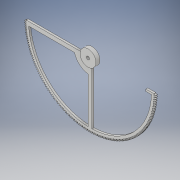
# Autodesk Inventor part: arm
Saved by Autodesk Inventor 2017 (Build 210142000, 142)
## iProperties
Created: 2016-11-23
Part Number: arm
Material: Generic
Document SubType Name: Modeling
Designer: cody
Density: 1 g/cm^3
Appearance: Default
Author: cody
Autodesk Inventor part; units mm, degrees
ref_plane "YZ Plane" through (0, 0, 0) normal (1, 0, 0) x (0, 1, 0)
ref_plane "XZ Plane" through (0, 0, 0) normal (0, 1, 0) x (-1, 0, 0)
ref_plane "XY Plane" through (0, 0, 0) normal (0, 0, 1) x (1, 0, 0)
sketch "Sketch1" plane through (0, 0, 0) normal (0, 0, 1) x (1, 0, 0)
  arc A0 (-50.8, 0) -> (50.8, 0) centre (0, 0) ccw
  line L0 (-50.8, 0) -> (50.8, 0)
  dimension "d0" = 101.6
  constraints: 2 end point, 2 point on circle, 1 centre point, 1 coincident, 1 horizontal
  measures "d0" diameter of A0
extrude "Extrusion1" add sketch "Sketch1" along normal blind 1.5875
sketch "Sketch2" plane through (0, 0, 1.5875) normal (0, 0, 1) x (1, 0, 0)
  arc A0 (-50.8, 0) -> (50.8, 0) centre (0, 0) ccw projected
  circle A1 centre (0, 0) radius 1.27
  circle A2 centre (0, 0) radius 6.35
  dimension "d4" = 2.54
  dimension "d5" = 12.7
  constraints: 2 centre point, 2 coincident
  measures "d4" diameter of A1
  measures "d5" diameter of A2
extrude "Extrusion2" add sketch "Sketch2" along normal mid plane 3.175
sketch "Sketch3" plane through (0, 0, 1.5875) normal (0, 0, 1) x (1, 0, 0)
  arc A0 (-6.35, 0) -> (6.35, 0) centre (0, 0) ccw projected
  line L0 (-6.35, 0) -> (-50.8, 0) projected
  arc A1 (-50.8, 0) -> (50.8, 0) centre (0, 0) ccw projected
  line L1 (50.8, 0) -> (6.35, 0) projected
  circle A2 centre (0, 0) radius 1.27 projected
  circle A3 centre (0, 0) radius 6.35 construction
  line L2 (1.5875, -12.6004) -> (1.5875, -48.8692)
  arc A4 (-12.2967, -3.175) -> (-1.5875, -12.6004) centre (0, 0) ccw
  arc A5 (1.5875, -12.6004) -> (12.7, 0) centre (0, 0) ccw
  arc A6 (-48.7918, -3.175) -> (-1.5875, -48.8692) centre (0, 0) ccw
  arc A7 (1.5875, -48.8692) -> (48.8692, -1.5875) centre (0, 0) ccw
  line L3 (0, 22.6021) -> (0, -65.0598) construction
  line L4 (-1.5875, -12.6004) -> (-1.5875, -48.8692)
  line L5 (44.45, -1.5875) -> (48.8692, -1.5875) construction
  line L6 (44.45, 0) -> (44.45, -1.5875)
  line L7 (44.45, -1.5875) -> (48.8692, -1.5875)
  line L8 (44.45, 0) -> (50.8, 0)
  line L9 (-49.7322, 0) -> (12.7, 0) construction
  line L10 (-76.619, 0) -> (71.9896, 0) construction
  line L11 (0, -3.175) -> (1.5875, -3.175)
  line L12 (-48.7918, -3.175) -> (-12.2967, -3.175)
  dimension "d13" = 44.45
  dimension "d34" = 3.175
  constraints: 22 end point, 8 point on circle, 5 centre point, 3 horizontal, 3 parallel, 3 point on line, 2 collinear, 1 coincident, 1 perpendicular, 1 vertical
  measures "d13" distance from line of A0.centre L6
  measures "d34" distance between parallel lines of L2 L4
extrude "Extrusion3" cut sketch "Sketch3" against normal blind 1.5875 contours L1 L6 L7 A7 L2 A5 | A4 L4 A6 L12
sketch "Sketch4" plane through (0, 0, 1.5875) normal (0, 0, 1) x (1, 0, 0)
  arc A0 (-50.8, 0) -> (50.8, 0) centre (0, 0) ccw projected
  line L0 (0, -55.6123) -> (0, -45.9148) construction
  line L1 (-0.381, -55.6123) -> (-0.381, -45.9148) construction
  line L2 (0.381, -55.6123) -> (0.381, -45.9148) construction
  line L3 (0.127, -55.6123) -> (0.127, -45.9148) construction
  line L4 (-0.127, -55.6123) -> (-0.127, -45.9148) construction
  arc A1 (0.1613, -51.9927) -> (0.381, -50.7986) centre (-2.4008, -50.9039) ccw
  line L5 (0.0444, -52.07) -> (-0.0443, -52.07)
  arc A2 (-0.381, -50.7986) -> (-0.1612, -51.9926) centre (2.4097, -50.9022) ccw
  arc A3 (0.0444, -52.07) -> (0.1613, -51.9927) centre (0.0444, -51.943) ccw
  arc A4 (-0.1612, -51.9926) -> (-0.0443, -52.07) centre (-0.0443, -51.943) ccw
  point P0 (0.127, -52.07)
  point P1 (-0.127, -52.07)
  dimension "d20" = 0.381
  dimension "d21" = 0.381
  dimension "d22" = 0.127
  dimension "d23" = 0.127
  dimension "d25" = 0.127
  constraints: 12 end point, 12 point on circle, 6 point on line, 4 centre point, 4 parallel, 4 tangent, 1 equal radius, 1 perpendicular, 1 vertical
  measures "d20" distance between parallel lines of L0 L1
  measures "d21" distance between parallel lines of L0 L2
  measures "d22" distance between parallel lines of L0 L3
  measures "d23" distance between parallel lines of L0 L4
  measures "d25" radius of A3
extrude "Extrusion4" add sketch "Sketch4" against normal blind 1.5875
pattern_circular "Circular Pattern1" count 121 over 178 about axis through (0, 0, -10) along (0, 0, 1) of "Extrusion4" both ways yes
sketch "Sketch6" plane through (0, 0, 3.175) normal (0, 0, 1) x (1, 0, 0)
  circle A0 centre (0, 0) radius 1.27 projected
  circle A1 centre (0, 0) radius 1.27
  constraints: 1 centre point, 1 coincident, 1 concentric
extrude "Extrusion5" cut sketch "Sketch6" along normal through all both and the other way through all
sketch "Sketch9" plane through (0, 0, 1.5875) normal (0, 0, 1) x (1, 0, 0)
  arc A0 (1.5875, -12.6004) -> (12.7, 0) centre (0, 0) ccw projected
  line L0 (12.7, 0) -> (6.35, 0) projected
  arc A1 (-6.35, 0) -> (6.35, 0) centre (0, 0) ccw projected
  arc A2 (-12.2967, -3.175) -> (-1.5875, -12.6004) centre (0, 0) ccw projected
  line L1 (1.5875, -6.1484) -> (1.5875, -12.6004)
  circle A3 centre (0, 0) radius 6.35
  circle A4 centre (0, 0) radius 12.7
  line L2 (0, 0) -> (12.7, 0)
  constraints: 4 end point, 2 coincident, 1 horizontal, 1 point on circle, 6 other
extrude "Extrusion6" cut sketch "Sketch9" against normal through all contours L1 A1 L0 A0
body "Solid1"
